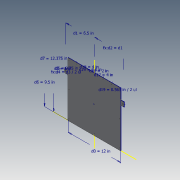
# Autodesk Inventor part: VP TRAY BASE SPACER
Saved by Autodesk Inventor 2020.3 (Build 243373000, 373)
## iProperties
RuleStatus: InUse
AfterDocSave0: file://Part Number Cleaner
Created: 2020-02-03
Material: Generic
Vendor: HHMI: JRC - ID&F
Document SubType Name: Modeling
Designer: arnoldj
Density: 1 g/cm^3
Appearance: Default
DESIGN DEPARTMENT: HHMI: JRC - ID&F
ALTERED ITEM PART NUMBER: N/A
ALTERED ITEM VENDOR: N/A
ALTERED ITEM DESCRIPTION: N/A
Author: arnoldj
Revision Number: 0
Autodesk Inventor part; units mm, degrees
ref_plane "YZ Plane" through (0, 0, 0) normal (1, 0, 0) x (0, 1, 0)
ref_plane "XZ Plane" through (0, 0, 0) normal (0, 1, 0) x (-1, 0, 0)
ref_plane "XY Plane" through (0, 0, 0) normal (0, 0, 1) x (1, 0, 0)
sketch "Sketch1" plane through (0, 0, 0) normal (0, 0, 1) x (1, 0, 0)
  line L0 (-240.03, 0) -> (240.03, 0) projected
  line L1 (0, 377.19) -> (0, -62.865) projected
  line L2 (152.4, 314.325) -> (-152.4, 314.325)
  line L3 (-152.4, 314.325) -> (-152.4, 0)
  line L4 (-152.4, 0) -> (152.4, 0)
  line L5 (152.4, 0) -> (152.4, 314.325)
  line L6 (152.4, 314.325) -> (-152.4, 0) construction
  line L7 (-152.4, 314.325) -> (152.4, 0) construction
  line L8 (-152.4, 228.6) -> (-171.45, 228.6)
  line L9 (-171.45, 228.6) -> (-171.45, 254)
  line L10 (-171.45, 254) -> (-152.4, 254)
  line L11 (-152.4, 254) -> (-152.4, 228.6)
  line L12 (152.4, 228.6) -> (171.45, 228.6)
  line L13 (171.45, 228.6) -> (171.45, 254)
  line L14 (171.45, 254) -> (152.4, 254)
  line L15 (152.4, 254) -> (152.4, 228.6)
  point P0 (0, 0)
  point P1 (0, 157.1625)
  point P2 (-165.1, 241.3)
  point P3 (165.1, 241.3)
  point P4 (101.6, 307.1749)
  point P5 (0, 307.1749)
  point P6 (-101.6, 307.1749)
  point P7 (-50.8, 307.1749)
  point P8 (50.8, 307.1749)
  dimension "d0" = 304.8
  dimension "d1" = 165.1
  dimension "d2" = 165.1
  dimension "d3" = 25.4
  dimension "d4" = 12.7
  dimension "d5" = 19.05
  dimension "d6" = 241.3
  dimension "d7" = 314.325
  dimension "d17" = 101.6
  dimension "d18" = 101.6
  dimension "d19" = 7.1501
  dimension "d29" = 50.8
  dimension "d30" = 50.8
  constraints: 28 end point, 6 horizontal alignment, 6 parallel, 4 point on line, 3 horizontal, 3 midpoint, 3 perpendicular, 2 equal length
  measures "d0" distance between parallel lines of L5 L3
  measures "d1" distance from line of point (-165.1, 241.3) L1
  measures "d2" distance from line of point (165.1, 241.3) L1
  measures "d3" distance of L8.end L9.end
  measures "d4" distance from line of point (-165.1, 241.3) L8
  measures "d5" distance of L9.end L10.end
  measures "d6" distance from line of L0 point (-165.1, 241.3)
  measures "d7" distance of L2.end L3.end
  measures "d17" distance from line of L1 point (101.6, 307.175)
  measures "d18" distance of point (0, 307.175) point (-101.6, 307.175)
  measures "d19" distance from line of point (101.6, 307.175) L2
  measures "d29" distance of point (0, 307.175) point (-50.8, 307.175)
  measures "d30" distance of point (0, 307.175) point (50.8, 307.175)
extrude "Extrusion1" add sketch "Sketch1" along normal blind 1.778
hole "Hole1" at (-165.1, 241.3, 0) at (165.1, 241.3, 0) direction (0, 0, 1) diameter 5.334 end through all clearance for "Flat Head Machine Screw (82)" size "#10" standard "Ansi Unified Screw Threads"
fillet "Fillet1" radius 3.175 2 edges at (152.4, 0, 0.889) (-152.4, 0, 0.889)
hole "Hole2" at (101.6, 307.1749, 0) at (0, 307.1749, 0) at (-101.6, 307.1749, 0) at (-50.8, 307.1749, 0) at (50.8, 307.1749, 0) direction (0, 0, 1) diameter 2.3876 end through all clearance for "Flat Head Machine Screw" size "M2" standard "Ansi Metric M Profile"
fillet "Fillet2" radius 6.35 10 edges at (152.4, 228.6, 0.889) (171.45, 228.6, 0.889) (171.45, 254, 0.889) (152.4, 254, 0.889) (152.4, 314.325, 0.889) (-152.4, 314.325, 0.889) (-152.4, 254, 0.889) (-171.45, 254, 0.889) (-171.45, 228.6, 0.889) (-152.4, 228.6, 0.889)
sketch "Sketch2" plane through (0, 0, 0) normal (0, 0, 1) x (1, 0, 0)
  line L0 (0, 377.19) -> (0, -62.865) projected
  line L1 (-152.4, 314.325) -> (152.4, 0) construction
  line L2 (152.4, 314.325) -> (-152.4, 0) construction
  line L3 (-146.05, 11.1125) -> (146.05, 11.1125) construction
  line L4 (146.05, 11.1125) -> (146.05, 303.2125) construction
  line L5 (146.05, 303.2125) -> (-146.05, 303.2125) construction
  line L6 (-146.05, 303.2125) -> (-146.05, 11.1125) construction
  line L7 (-146.05, 11.1125) -> (146.05, 303.2125) construction
  line L8 (146.05, 11.1125) -> (-146.05, 303.2125) construction
  point P0 (0, 0)
  point P1 (0, 157.1625)
  point P2 (0, 303.2125)
  point P3 (-146.05, 157.1625)
  point P4 (0, 11.1125)
  point P5 (0, 157.1625)
  point P6 (146.05, 157.1625)
  dimension "d31" = 292.1
  dimension "d32" = 292.1
  constraints: 12 end point, 7 midpoint, 2 parallel, 1 coincident, 1 horizontal, 1 perpendicular
  measures "d31" distance of L4.end L5.end
  measures "d32" distance of L3.end L4.end
hole "Hole3" at (-146.05, 11.1125, 0) at (146.05, 11.1125, 0) at (146.05, 303.2125, 0) at (-146.05, 303.2125, 0) at (146.05, 157.1625, 0) at (0, 11.1125, 0) at (0, 157.1625, 0) at (-146.05, 157.1625, 0) at (0, 303.2125, 0) direction (0, 0, 1) diameter 2.4384 end through all countersink diameter 4.3688 countersink angle 100 clearance for "Flat Head Machine Screw (100)" size "#2" standard "Ansi Unified Screw Threads"
equation "\"d2\" = d1"
equation "\"d4\" = 0.5 * d3"
body "Solid1"
